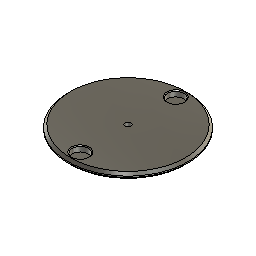
Tachometer Disk  v4 (Autodesk Fusion 360 design; units mm, degrees)
Autodesk Fusion 360 part; units mm, degrees
sketch "Sketch1" plane through (0, 0, 0) normal (0, 0, 1) x (1, 0, 0)
  circle A0 centre (0, 0) radius 30
  circle A1 centre (0, 23.95) radius 4.05
  line L0 (-30, 0) -> (30, 0)
  circle A2 centre (0, -23.95) radius 4.05
  circle A3 centre (0, 0) radius 1.45
  dimension "d1" = 60
  dimension "d2" = 8.1
  dimension "d3" = 2
  dimension "d4" = 2.9
  constraint coincident A0.centre A3.centre
  constraint vertical A0.centre A1.centre
  constraint coincident A0 L0.start
  constraint coincident A0 L0.end
  constraint horizontal L0
  constraint symmetric A1 L0 A2
  constraint coincident A0.centre L0
  constraint concentric A0 A3
  measures "d1" diameter of A0
  measures "d2" diameter of A1
  measures "d4" diameter of A3
extrude "Extrude1" add sketch "Sketch1" against normal blind 3 contours A0 L0 A3 | A0 L0 A3 | A1 | A2
extrude "Extrude2" cut sketch "Sketch1" against normal blind 2.8 contours A1 | A2
chamfer "Chamfer1" distance 1.2 angle 45 2 edges at (-27.9698, -10.8485, 0) (-27.9698, 10.8485, -3)
chamfer "Chamfer2" distance 0.4 angle 45 2 edges at (-3.7759, -22.4855, 0) (-3.7759, 25.4145, 0)
